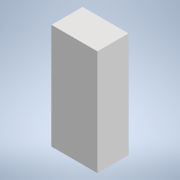
# Autodesk Inventor part: new battery
Saved by Autodesk Inventor 2022.3 (Build 263350030, 350C)
## iProperties
Created: 2024-10-06
Part Number: new battery
Material: Generic
Document SubType Name: Modeling
Designer: Zhong
Density: 1 g/cm^3
Appearance: Default
Author: Zhong
Autodesk Inventor part; units mm, degrees
ref_plane "YZ Plane" through (0, 0, 0) normal (1, 0, 0) x (0, 1, 0)
ref_plane "XZ Plane" through (0, 0, 0) normal (0, 1, 0) x (-1, 0, 0)
ref_plane "XY Plane" through (0, 0, 0) normal (0, 0, 1) x (1, 0, 0)
sketch "Sketch1" plane through (0, 0, 0) normal (0, 0, 1) x (1, 0, 0)
  line L0 (17, 39) -> (-17, 39)
  line L1 (-17, 39) -> (-17, -39)
  line L2 (-17, -39) -> (17, -39)
  line L3 (17, -39) -> (17, 39)
  line L4 (17, 0) -> (-17, 0) construction
  line L5 (0, 39) -> (0, -39) construction
  point P0 (0, 0)
  point P1 (0, 0)
  dimension "d0" = 34
  dimension "d1" = 78
  constraints: 12 end point, 5 midpoint, 2 parallel, 1 coincident, 1 horizontal, 1 perpendicular
  measures "d0" distance of L2.end L1.end
  measures "d1" distance of L1.end L0.end
extrude "Extrusion1" add sketch "Sketch1" along normal blind 23
body "Solid1"
